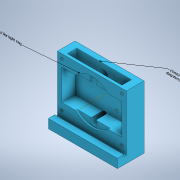
# Autodesk Inventor part: 2020PiZeroCameraLightRingMount
Saved by Autodesk Inventor 2020.2 (Build 242310000, 310)
## iProperties
Created: 2019-10-10
Part Number: 2020PiZeroCameraLightRingMount
Material: PC/ABS Plastic
Document SubType Name: Modeling
Designer: steele
Density: 0.357273 g/cm^3
Appearance: Turquoise
Author: steele
Autodesk Inventor part; units mm, degrees
ref_plane "YZ Plane" through (0, 0, 0) normal (1, 0, 0) x (0, 1, 0)
ref_plane "XZ Plane" through (0, 0, 0) normal (0, 1, 0) x (-1, 0, 0)
ref_plane "XY Plane" through (0, 0, 0) normal (0, 0, 1) x (1, 0, 0)
sketch "Sketch1" plane through (0, 0, 0) normal (0, 0, 1) x (1, 0, 0)
  line L0 (-48.5775, -37.85) -> (48.5775, -37.85)
  line L1 (48.5775, -37.85) -> (48.5775, 37.85)
  line L2 (48.5775, 37.85) -> (-48.5775, 37.85)
  line L3 (-48.5775, 37.85) -> (-48.5775, -37.85)
  line L4 (-48.5775, -37.85) -> (48.5775, 37.85) construction
  line L5 (48.5775, -37.85) -> (-48.5775, 37.85) construction
  point P0 (0, 0)
  dimension "majorPartWidth" = 97.155
  dimension "majorPartHeight" = 75.7
  constraints: 12 end point, 2 midpoint, 2 parallel, 1 horizontal, 1 perpendicular
  measures "majorPartWidth" distance of L0.start L0.end
  measures "majorPartHeight" distance of L1.end L0.end
extrude "Extrusion1" add sketch "Sketch1" against normal blind 24.725
sketch "Sketch2" plane through (0, 0, 0) normal (0, 0, 1) x (1, 0, 0)
  line L0 (-42.2275, -21.59) -> (42.2275, -21.59)
  line L1 (42.2275, -21.59) -> (42.2275, 21.59)
  line L2 (42.2275, 21.59) -> (-42.2275, 21.59)
  line L3 (-42.2275, 21.59) -> (-42.2275, -21.59)
  line L4 (-42.2275, -21.59) -> (42.2275, 21.59) construction
  line L5 (42.2275, -21.59) -> (-42.2275, 21.59) construction
  point P0 (0, 0)
  dimension "holeForPiCaseWidth" = 84.455
  dimension "holeForPiCaseHeight" = 43.18
  constraints: 12 end point, 2 midpoint, 2 parallel, 1 horizontal, 1 perpendicular
  measures "holeForPiCaseWidth" distance of L0.start L0.end
  measures "holeForPiCaseHeight" distance of L1.end L0.end
extrude "Extrusion2" cut sketch "Sketch2" against normal blind 18.375
sketch "Sketch3" plane through (0, 0, 0) normal (0, 0, 1) x (1, 0, 0)
  circle A0 centre (0, 0) radius 31.5
  circle A1 centre (0, 0) radius 18.5
  dimension "lightRingHoleExteriorDiam" = 63
  dimension "lightRingHoleInteriorDiam" = 37
  constraints: 2 centre point, 2 coincident
  measures "lightRingHoleExteriorDiam" diameter of A0
  measures "lightRingHoleInteriorDiam" diameter of A1
extrude "Extrusion3" cut sketch "Sketch3" against normal blind 2.5
sketch "Sketch4" plane through (0, 0, -2.5) normal (0, 0, 1) x (1, 0, 0)
  circle A0 centre (0, 0) radius 25.4466 construction
  circle A1 centre (0, 25.4466) radius 5
  circle A2 centre (0, -25.4466) radius 5
  dimension "holeForLightRingWires" = 10
  dimension "d13" = 10
  constraints: 3 centre point, 2 point on circle, 1 coincident
  measures "holeForLightRingWires" diameter of A1
  measures "d13" diameter of A2
extrude "Extrusion4" cut sketch "Sketch4" against normal through all
sketch "Sketch6" plane through (-48.5775, -37.85, 0) normal (0, -1, 0) x (1, 0, 0)
  line L0 (0, -24.725) -> (97.155, -24.725) projected
  line L1 (0, -24.725) -> (97.155, -24.725)
  line L2 (97.155, -24.725) -> (97.155, 12.7)
  line L3 (97.155, 12.7) -> (0, 12.7)
  line L4 (0, 12.7) -> (0, -24.725)
  point P0 (48.5775, 0)
  dimension "baseWidth" = 97.155
  dimension "baseDepth" = 37.425
  constraints: 8 end point, 2 parallel, 1 horizontal, 1 perpendicular
  measures "baseWidth" distance of L2.end L3.end
  measures "baseDepth" distance of L1.end L2.end
extrude "Extrusion6" add sketch "Sketch6" along normal blind 12.7
sketch "Sketch7" plane through (-48.5775, 37.85, 0) normal (0, 1, 0) x (1, 0, 0)
  line L0 (97.155, 0) -> (0, 0) construction
  line L1 (0, 0) -> (0, 24.725) construction
  line L2 (10.16, 3.77) -> (86.995, 3.77)
  line L3 (86.995, 3.77) -> (86.995, 17.105)
  line L4 (86.995, 17.105) -> (10.16, 17.105)
  line L5 (10.16, 17.105) -> (10.16, 3.77)
  line L6 (10.16, 3.77) -> (86.995, 17.105) construction
  line L7 (86.995, 3.77) -> (10.16, 17.105) construction
  line L8 (45.3952, 18.375) -> (45.3952, 2.5) projected
  point P0 (48.5775, 0)
  point P1 (48.5775, 10.4375)
  dimension "y" = 10.4375
  dimension "Y" = 48.5775
  dimension "piWireDepth" = 13.335
  dimension "piWireWidth" = 76.835
  constraints: 12 end point, 2 midpoint, 2 parallel, 2 perpendicular
  measures "y" distance from line of point (48.577, 10.438) L0
  measures "Y" distance from line of point (48.577, 10.438) L1
  measures "piWireDepth" distance of L4.end L2.start
  measures "piWireWidth" distance of L3.end L4.end
extrude "Extrusion7" cut sketch "Sketch7" against normal up to next
sketch "Sketch8" plane through (-48.5775, 37.85, -24.725) normal (-1, 0, 0) x (0, 0, 1)
  line L0 (24.725, -75.7) -> (24.725, 0) projected
  line L1 (24.725, -75.7) -> (28.535, -75.7)
  line L2 (28.535, -75.7) -> (28.535, -78.24)
  line L3 (28.535, -78.24) -> (24.725, -78.24)
  line L4 (24.725, -78.24) -> (24.725, -75.7)
  point P0 (24.725, -37.85)
  dimension "d30" = 3.81
  dimension "d31" = 2.54
  constraints: 8 end point, 2 parallel, 1 horizontal, 1 perpendicular
  measures "d30" distance of L2.end L3.end
  measures "d31" distance of L1.end L2.end
extrude "Extrusion8" cut sketch "Sketch8" against normal through all
sketch "Sketch9" plane through (0, 0, 0) normal (0, 0, 1) x (1, 0, 0)
  point P0 (-42.2275, 31.5)
  point P1 (42.2275, 31.5)
  point P2 (42.2275, -31.5)
  point P3 (-42.2275, -31.5)
hole "Hole1" at (-42.2275, 31.5, 0) at (42.2275, 31.5, 0) at (42.2275, -31.5, 0) at (-42.2275, -31.5, 0) direction (0, 0, -1) diameter 3.683 depth 14.986 tip angle 120 thread size "10-24 UNC" class "2B" standard "ANSI Unified Screw Threads"
sketch "Sketch10" plane through (0, 0, -24.725) normal (0, 0, -1) x (-1, 0, 0)
  point P0 (-39.0525, 23.7022)
  point P1 (-16.8275, 23.7022)
  point P2 (-16.8275, -11.2228)
  point P3 (-39.0525, -11.2228)
hole "Hole3" at (39.0525, 23.7022, -24.725) at (16.8275, 23.7022, -24.725) at (16.8275, -11.2228, -24.725) at (39.0525, -11.2228, -24.725) direction (0, 0, 1) diameter 3.9624 depth 11.9507 tip angle 120 thread size "10-32 UNF" class "2B" standard "ANSI Unified Screw Threads"
equation "\"majorPartWidth\" = holeForPiCaseWidth + 2 * minWallThickness"
equation "\"majorPartHeight\" = lightRingHoleExteriorDiam + 2 * minWallThickness"
equation "\"majorPartDepth\" = holeForPiCaseDepth + minWallThickness"
equation "\"holeForPiCaseWidth\" = piCaseWidth + 2 * caseGap"
equation "\"holeForPiCaseHeight\" = piCaseHeight + 2 * caseGap"
equation "\"holeForPiCaseDepth\" = PiCaseDepth + depthForLightRing"
equation "\"lightRingHoleExteriorDiam\" = lightRingExteriorDiam + lightRingEdgeSpacing"
equation "\"lightRingHoleInteriorDiam\" = lightRingInterorDiam - lightRingEdgeSpacing"
equation "\"d13\" = holeForLightRingWires"
equation "\"baseWidth\" = majorPartWidth"
equation "\"y\" = 0.5 * PiCaseDepth + depthForLightRing"
equation "\"Y\" = 0.5 * majorPartWidth"
equation "\"minWallThickness\" = 6.35"
equation "\"lightRingEdgeSpacing\" = 3"
equation "\"lightRingExteriorDiam\" = 60"
equation "\"lightRingInterorDiam\" = 40"
equation "\"caseGap\" = 2.54"
equation "\"piCaseWidth\" = 79.375"
equation "\"piCaseHeight\" = 38.1"
equation "\"PiCaseDepth\" = 15.875"
equation "\"depthForLightRing\" = 2.5"
body "Solid1"
